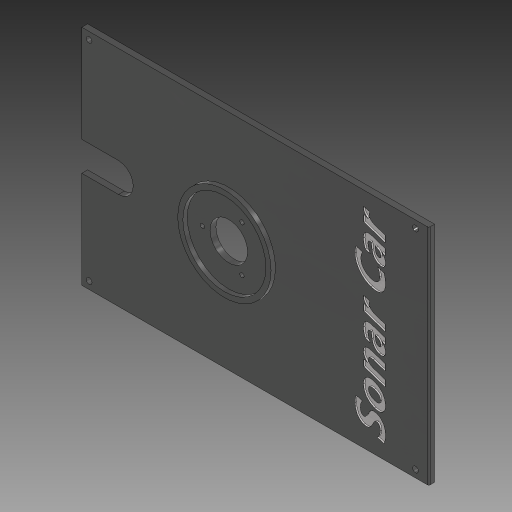
# Autodesk Inventor part: box-top
Saved by Autodesk Inventor 2023 (Build 270158000, 158)
## iProperties
Created: 2024-02-02
Part Number: box-top
Material: Všeobecné
Document SubType Name: Modeling
Designer: matej
Mass: 17.4288 g
Surface Area: 187.276 cm^2
Volume: 17.4288 cm^3
Density: 1 g/cm^3
Appearance: Tmavě šedá
Author: matej
## iProperties of the stored document box-top_3D tisk.ipt
Created: 2024-02-13
Part Number: box-top_3D tisk
Material: Všeobecné
Document SubType Name: Modeling
Designer: zak
Density: 1 g/cm^3
Appearance: Výchozí
Mass: 17.4407 g
Surface Area: 187.376 cm^2
Volume: 17.4407 cm^3
Author: zak
Autodesk Inventor part; units mm, degrees
ref_plane "YZ Plane" through (0, 0, 0) normal (1, 0, 0) x (0, 1, 0)
ref_plane "XZ Plane" through (0, 0, 0) normal (0, 1, 0) x (-1, 0, 0)
ref_plane "XY Plane" through (0, 0, 0) normal (0, 0, 1) x (1, 0, 0)
sketch "Náčrt1" plane through (0, 0, 0) normal (0, 0, 1) x (1, 0, 0)
  line L0 (60, 40) -> (-60, 40)
  line L1 (-60, 40) -> (-60, -40)
  line L2 (-60, -40) -> (60, -40)
  line L3 (60, -40) -> (60, 40)
  line L4 (60, 40) -> (-60, -40) construction
  line L5 (-60, 40) -> (60, -40) construction
  line L6 (58, 38) -> (53, 38)
  line L7 (53, 38) -> (53, 33)
  line L8 (53, 33) -> (58, 33)
  line L9 (58, 33) -> (58, 38)
  line L10 (53, 38) -> (58, 33) construction
  line L11 (58, 38) -> (53, 33) construction
  circle A0 centre (55.5, 35.5) radius 1
  line L12 (58, -33) -> (53, -33)
  line L13 (53, -33) -> (53, -38)
  line L14 (53, -38) -> (58, -38)
  circle A1 centre (55.5, -35.5) radius 1
  line L15 (53, -33) -> (58, -38) construction
  line L16 (58, -33) -> (53, -38) construction
  line L17 (58, -38) -> (58, -33)
  line L18 (-53, 38) -> (-58, 38)
  line L19 (-58, 38) -> (-58, 33)
  line L20 (-58, 33) -> (-53, 33)
  circle A2 centre (-55.5, 35.5) radius 1
  line L21 (-58, 38) -> (-53, 33) construction
  line L22 (-53, 38) -> (-58, 33) construction
  line L23 (-53, 33) -> (-53, 38)
  line L24 (-53, -33) -> (-58, -33)
  line L25 (-58, -33) -> (-58, -38)
  line L26 (-58, -38) -> (-53, -38)
  circle A3 centre (-55.5, -35.5) radius 1
  line L27 (-58, -33) -> (-53, -38) construction
  line L28 (-53, -33) -> (-58, -38) construction
  line L29 (-53, -38) -> (-53, -33)
  line L30 (-58, 38) -> (60, 38)
  line L31 (60, 38) -> (60, -38)
  line L32 (60, -38) -> (-58, -38)
  line L33 (-58, -38) -> (-58, 38)
  point P0 (0, 0)
  dimension "d0" = 120
  dimension "d1" = 80
  dimension "d2" = 5
  dimension "d3" = 5
  dimension "d4" = 2
  dimension "d5" = 2.5
  dimension "d6" = 2
  dimension "d7" = 2
  dimension "d10" = 71
  dimension "d13" = 111
  constraints: 68 end point, 6 parallel, 4 centre point, 4 horizontal, 3 midpoint, 3 perpendicular, 1 point on line, 1 vertical, 39 other
  measures "d0" distance of L0.start L0.end
  measures "d1" distance of L2.end L0.start
  measures "d2" distance of L8.end L7.end
  measures "d3" distance of L7.end L6.end
  measures "d4" diameter of A0
  measures "d5" distance from line of L8 A0.centre
  measures "d6" distance between parallel lines of L0 L6
  measures "d7" distance between parallel lines of L3 L9
  measures "d10" distance of L6.start L12.start
  measures "d13" distance of L6.start L18.start
extrude "Vysunutí1" add sketch "Náčrt1" along normal blind 2 contours L3 L32 L17 L12 L13 L29 L24 L33 L20 L23 L30 L7 L8 L9 | L9 L8 L7 L6 | L14 L13 L12 L17 | L23 L20 L19 L18 | L26 L25 L24 L29
sketch "Náčrt2" plane through (0, 0, 2) normal (0, 0, 1) x (1, 0, 0)
  circle A0 centre (-8, 0) radius 6.4
  line L0 (-58, 38) -> (-58, -38) projected
  point P0 (0, 0)
  dimension "d18" = 12.8
  dimension "d25" = 50
  constraints: 1 centre point
  measures "d18" diameter of A0
  measures "d25" distance from line of L0 A0.centre
extrude "Vysunutí2" cut sketch "Náčrt2" against normal through all
sketch "Náčrt3" plane through (0, 0, 2) normal (0, 0, 1) x (1, 0, 0)
  circle A0 centre (-45.5, 0) radius 5
  line L0 (-58, 38) -> (-58, -38) projected
  line L1 (-70.5, -5) -> (-45.5, -5)
  line L2 (-45.5, -5) -> (-45.5, 5)
  line L3 (-45.5, 5) -> (-70.5, 5)
  line L4 (-70.5, 5) -> (-70.5, -5)
  line L5 (-70.5, -5) -> (-45.5, 5) construction
  line L6 (-45.5, -5) -> (-70.5, 5) construction
  point P0 (0, 0)
  point P1 (-58, 0)
  point P2 (-45.5, -5)
  point P3 (-45.5, 5)
  dimension "d21" = 12.5
  dimension "d22" = 10
  dimension "d43" = 10
  dimension "d44" = 25
  constraints: 12 end point, 3 midpoint, 2 parallel, 1 centre point, 1 horizontal, 1 perpendicular
  measures "d21" distance from line of L0 A0.centre
  measures "d22" diameter of A0
  measures "d43" distance of L1.end L2.end
  measures "d44" distance between parallel lines of L4 L2
extrude "Vysunutí3" cut sketch "Náčrt3" against normal through all
sketch "Náčrt4" plane through (0, 0, 2) normal (0, 0, 1) x (1, 0, 0)
  circle A0 centre (-8, 0) radius 6.4 projected
  circle A1 centre (-8, 0) radius 14.125
  circle A2 centre (-8, 0) radius 15.875
  point P0 (0, 0)
  dimension "d26" = 28.25
  dimension "d27" = 31.75
  constraints: 2 centre point, 2 coincident
  measures "d26" diameter of A1
  measures "d27" diameter of A2
extrude "Vysunutí4" add sketch "Náčrt4" along normal blind 1.5 contours A2
sketch "Náčrt5" plane through (0, 0, 2) normal (0, 0, 1) x (1, 0, 0)
  circle A0 centre (-17, 0) radius 0.75
  circle A1 centre (-8, 0) radius 6.4 projected
  circle A2 centre (-3.5, -7.7942) radius 0.75
  circle A3 centre (-3.5, 7.7942) radius 0.75
  point P0 (0, 0)
  dimension "d31" = 1.5
  dimension "d34" = 360
  dimension "d36" = 9
  constraints: 3 centre point, 2 coincident, 8 other
  measures "d31" diameter of A0
  measures "d36" distance of A1.centre A0.centre
extrude "Vysunutí5" cut sketch "Náčrt5" against normal through all contours A0 | A2 | A3
sketch "Náčrt6" plane through (0, 0, 2) normal (0, 0, 1) x (1, 0, 0)
  line L0 (34.9532, -34.0683) -> (34.9532, 34.0683) construction
  line L1 (34.9532, 34.0683) -> (55, 34.0683) construction
  line L2 (55, 34.0683) -> (55, -34.0683) construction
  line L3 (55, -34.0683) -> (34.9532, -34.0683) construction
  line L4 (60, -38) -> (60, 38) projected
  line L5 (44.7398, -33.252) -> (42.5042, -32.4913)
  spline S0 degree 2 poles (42.5042, -32.4913) (43.0144, -32.0646) (43.5246, -30.8123) (43.5246, -30.0887) knots 0 0 0 1 2 2 2
  spline S1 degree 2 poles (43.5246, -30.0887) (43.5246, -29.662) (43.3669, -28.9756) (43.0979, -28.4561) (42.7268, -28.1221) (42.5135, -28.0479) knots 0 0 0 1 2 3 4 4 4
  spline S2 degree 2 poles (42.5135, -28.0479) (42.2166, -27.9459) (41.7621, -28.1221) (41.3632, -28.5767) (41.0014, -29.2446) (40.8159, -29.6435) knots 0 0 0 1 2 3 4 4 4
  spline S3 degree 2 poles (40.8159, -29.6435) (40.3242, -30.6453) (38.9235, -31.3225) (37.9216, -30.9793) knots 0 0 0 1 2 2 2
  spline S4 degree 2 poles (37.9216, -30.9793) (37.1424, -30.7103) (36.02, -29.7084) (35.2871, -28.3819) (34.9532, -26.842) (34.9532, -26.0442) knots 0 0 0 1 2 3 4 4 4
  spline S5 degree 2 poles (34.9532, -26.0442) (34.9532, -25.265) (35.1387, -24.1147) (35.3335, -23.6787) knots 0 0 0 1 2 2 2
  line L6 (35.3335, -23.6787) -> (37.4207, -24.3837)
  spline S6 degree 2 poles (37.4207, -24.3837) (37.2445, -24.5785) (36.9754, -25.0795) (36.8085, -25.6453) (36.725, -26.239) (36.725, -26.5173) knots 0 0 0 1 2 3 4 4 4
  spline S7 degree 2 poles (36.725, -26.5173) (36.725, -26.9069) (36.8641, -27.5841) (37.1331, -28.1036) (37.5042, -28.4654) (37.7361, -28.5489) knots 0 0 0 1 2 3 4 4 4
  spline S8 degree 2 poles (37.7361, -28.5489) (37.9866, -28.6323) (38.3855, -28.5025) (38.738, -28.1314) (39.0812, -27.547) (39.2574, -27.1759) knots 0 0 0 1 2 3 4 4 4
  spline S9 degree 2 poles (39.2574, -27.1759) (39.5079, -26.6565) (40.0738, -25.8958) (40.7881, -25.4505) (41.7064, -25.4041) (42.3094, -25.6082) knots 0 0 0 1 2 3 4 4 4
  spline S10 degree 2 poles (42.3094, -25.6082) (43.1443, -25.8958) (44.2853, -26.9162) (44.9903, -28.2427) (45.2964, -29.7919) (45.2964, -30.5897) knots 0 0 0 1 2 3 4 4 4
  spline S11 degree 2 poles (45.2964, -30.5897) (45.2964, -31.4153) (45.0181, -32.8067) (44.7398, -33.252) knots 0 0 0 1 2 2 2
  spline S12 degree 2 poles (45.2964, -21.7863) (45.2964, -23.5767) (43.2927, -24.9403) (41.5766, -24.3559) knots 0 0 0 1 2 2 2
  spline S13 degree 2 poles (41.5766, -24.3559) (39.8048, -23.7529) (37.801, -20.9515) (37.801, -19.1426) knots 0 0 0 1 2 2 2
  spline S14 degree 2 poles (37.801, -19.1426) (37.801, -17.3708) (39.8048, -16.0257) (41.4467, -16.5823) knots 0 0 0 1 2 2 2
  spline S15 degree 2 poles (41.4467, -16.5823) (43.2278, -17.1852) (45.2964, -19.9774) (45.2964, -21.7863) knots 0 0 0 1 2 2 2
  spline S16 degree 2 poles (39.4894, -19.7641) (39.4894, -20.5433) (40.5654, -21.7771) (41.5487, -22.111) knots 0 0 0 1 2 2 2
  spline S17 degree 2 poles (41.5487, -22.111) (43.6081, -22.8067) (43.6081, -21.1463) knots 0 0 0 1 1 1
  spline S18 degree 2 poles (43.6081, -21.1463) (43.6081, -19.56) (41.4931, -18.8457) knots 0 0 0 1 1 1
  spline S19 degree 2 poles (41.4931, -18.8457) (39.4894, -18.1685) (39.4894, -19.7641) knots 0 0 0 1 1 1
  line L7 (45.1202, -9.5043) -> (45.1202, -11.7028)
  line L8 (45.1202, -11.7028) -> (41.1498, -10.3578)
  spline S20 degree 2 poles (41.1498, -10.3578) (39.4894, -9.7919) (39.4894, -10.9793) knots 0 0 0 1 1 1
  spline S21 degree 2 poles (39.4894, -10.9793) (39.4894, -11.5451) (40.3706, -12.5841) (41.0478, -12.816) knots 0 0 0 1 2 2 2
  line L9 (41.0478, -12.816) -> (45.1202, -14.1982)
  line L10 (45.1202, -14.1982) -> (45.1202, -16.406)
  line L11 (45.1202, -16.406) -> (37.9773, -13.9756)
  line L12 (37.9773, -13.9756) -> (37.9773, -11.7771)
  line L13 (37.9773, -11.7771) -> (39.109, -12.1574)
  line L14 (39.109, -12.1574) -> (39.109, -12.1296)
  spline S22 degree 2 poles (39.109, -12.1296) (37.801, -10.8958) (37.801, -9.393) knots 0 0 0 1 1 1
  spline S23 degree 2 poles (37.801, -9.393) (37.801, -7.0182) (40.751, -8.0201) knots 0 0 0 1 1 1
  line L15 (40.751, -8.0201) -> (45.1202, -9.5043)
  line L16 (45.1202, -1.8142) -> (45.1202, -3.9014)
  line L17 (45.1202, -3.9014) -> (44.0905, -3.5581)
  line L18 (44.0905, -3.5581) -> (44.0905, -3.586)
  spline S24 degree 2 poles (44.0905, -3.586) (45.2964, -4.7084) (45.2964, -6.1184) knots 0 0 0 1 1 1
  spline S25 degree 2 poles (45.2964, -6.1184) (45.2964, -7.1574) (44.1183, -7.9459) (43.135, -7.6119) knots 0 0 0 1 2 2 2
  spline S26 degree 2 poles (43.135, -7.6119) (41.0571, -6.9069) (40.7324, -4.3374) knots 0 0 0 1 1 1
  line L19 (40.7324, -4.3374) -> (40.4727, -2.3058)
  spline S27 degree 2 poles (40.4727, -2.3058) (39.3038, -1.9162) (39.3038, -3.1778) knots 0 0 0 1 1 1
  spline S28 degree 2 poles (39.3038, -3.1778) (39.3038, -4.458) (40.0645, -5.868) knots 0 0 0 1 1 1
  line L20 (40.0645, -5.868) -> (38.404, -5.3021)
  spline S29 degree 2 poles (38.404, -5.3021) (38.1628, -4.7641) (37.801, -3.0387) (37.801, -2.3893) knots 0 0 0 1 2 2 2
  spline S30 degree 2 poles (37.801, -2.3893) (37.801, 0.6719) (40.853, -0.367) knots 0 0 0 1 1 1
  line L21 (40.853, -0.367) -> (45.1202, -1.8142)
  line L22 (42.2166, -2.8995) -> (41.7343, -2.7418)
  line L23 (41.7343, -2.7418) -> (41.9012, -4.0962)
  spline S31 degree 2 poles (41.9012, -4.0962) (42.0404, -5.2186) (42.8753, -5.4969) knots 0 0 0 1 1 1
  spline S32 degree 2 poles (42.8753, -5.4969) (43.2463, -5.6268) (43.7287, -5.265) (43.7287, -4.8197) knots 0 0 0 1 2 2 2
  spline S33 degree 2 poles (43.7287, -4.8197) (43.7287, -4.1982) (42.8753, -3.1221) (42.2166, -2.8995) knots 0 0 0 1 2 2 2
  spline S34 degree 2 poles (39.9625, 6.3398) (39.7491, 6.0151) (39.7491, 5.4864) knots 0 0 0 1 1 1
  spline S35 degree 2 poles (39.7491, 5.4864) (39.7491, 4.7721) (40.8066, 3.6033) (41.7064, 3.2972) knots 0 0 0 1 2 2 2
  line L24 (41.7064, 3.2972) -> (45.1202, 2.1376)
  line L25 (45.1202, 2.1376) -> (45.1202, -0.0702)
  line L26 (45.1202, -0.0702) -> (37.9773, 2.3602)
  line L27 (37.9773, 2.3602) -> (37.9773, 4.5587)
  line L28 (37.9773, 4.5587) -> (39.3038, 4.1135)
  line L29 (39.3038, 4.1135) -> (39.3038, 4.1413)
  spline S36 degree 2 poles (39.3038, 4.1413) (37.8474, 5.1524) (37.8474, 6.5161) knots 0 0 0 1 1 1
  spline S37 degree 2 poles (37.8474, 6.5161) (37.8474, 6.8686) (37.9309, 7.0356) knots 0 0 0 1 1 1
  line L30 (37.9309, 7.0356) -> (39.9625, 6.3398)
  spline S38 degree 2 poles (44.7676, 17.0634) (45.2964, 15.7925) (45.2964, 14.03) knots 0 0 0 1 1 1
  spline S39 degree 2 poles (45.2964, 14.03) (45.2964, 11.7294) (42.5877, 10.004) (40.3335, 10.774) knots 0 0 0 1 2 2 2
  spline S40 degree 2 poles (40.3335, 10.774) (37.9309, 11.5903) (34.9532, 15.5699) (34.9532, 17.9354) knots 0 0 0 1 2 2 2
  spline S41 degree 2 poles (34.9532, 17.9354) (34.9532, 19.401) (35.315, 20.273) knots 0 0 0 1 1 1
  line L31 (35.315, 20.273) -> (37.4856, 19.5402)
  spline S42 degree 2 poles (37.4856, 19.5402) (36.892, 18.7424) (36.892, 17.453) knots 0 0 0 1 1 1
  spline S43 degree 2 poles (36.892, 17.453) (36.892, 16.043) (38.6638, 13.7146) (40.1758, 13.2044) knots 0 0 0 1 2 2 2
  spline S44 degree 2 poles (40.1758, 13.2044) (41.6229, 12.7035) (43.3484, 13.7517) (43.3484, 15.1339) knots 0 0 0 1 2 2 2
  spline S45 degree 2 poles (43.3484, 15.1339) (43.3484, 16.4511) (42.7083, 17.7684) knots 0 0 0 1 1 1
  line L32 (42.7083, 17.7684) -> (44.7676, 17.0634)
  line L33 (45.1202, 24.4196) -> (45.1202, 22.3324)
  line L34 (45.1202, 22.3324) -> (44.0905, 22.6756)
  line L35 (44.0905, 22.6756) -> (44.0905, 22.6478)
  spline S46 degree 2 poles (44.0905, 22.6478) (45.2964, 21.5254) (45.2964, 20.1153) knots 0 0 0 1 1 1
  spline S47 degree 2 poles (45.2964, 20.1153) (45.2964, 19.0764) (44.1183, 18.2879) (43.135, 18.6218) knots 0 0 0 1 2 2 2
  spline S48 degree 2 poles (43.135, 18.6218) (41.0571, 19.3268) (40.7324, 21.8964) knots 0 0 0 1 1 1
  line L36 (40.7324, 21.8964) -> (40.4727, 23.9279)
  spline S49 degree 2 poles (40.4727, 23.9279) (39.3038, 24.3176) (39.3038, 23.056) knots 0 0 0 1 1 1
  spline S50 degree 2 poles (39.3038, 23.056) (39.3038, 21.7758) (40.0645, 20.3658) knots 0 0 0 1 1 1
  line L37 (40.0645, 20.3658) -> (38.404, 20.9317)
  spline S51 degree 2 poles (38.404, 20.9317) (38.1628, 21.4697) (37.801, 23.1951) (37.801, 23.8445) knots 0 0 0 1 2 2 2
  spline S52 degree 2 poles (37.801, 23.8445) (37.801, 26.9057) (40.853, 25.8667) knots 0 0 0 1 1 1
  line L38 (40.853, 25.8667) -> (45.1202, 24.4196)
  line L39 (42.2166, 23.3343) -> (41.7343, 23.492)
  line L40 (41.7343, 23.492) -> (41.9012, 22.1376)
  spline S53 degree 2 poles (41.9012, 22.1376) (42.0404, 21.0151) (42.8753, 20.7369) knots 0 0 0 1 1 1
  spline S54 degree 2 poles (42.8753, 20.7369) (43.2463, 20.607) (43.7287, 20.9688) (43.7287, 21.414) knots 0 0 0 1 2 2 2
  spline S55 degree 2 poles (43.7287, 21.414) (43.7287, 22.0356) (42.8753, 23.1116) (42.2166, 23.3343) knots 0 0 0 1 2 2 2
  spline S56 degree 2 poles (39.9625, 32.5736) (39.7491, 32.2489) (39.7491, 31.7202) knots 0 0 0 1 1 1
  spline S57 degree 2 poles (39.7491, 31.7202) (39.7491, 31.0059) (40.8066, 29.837) (41.7064, 29.5309) knots 0 0 0 1 2 2 2
  line L41 (41.7064, 29.5309) -> (45.1202, 28.3714)
  line L42 (45.1202, 28.3714) -> (45.1202, 26.1636)
  line L43 (45.1202, 26.1636) -> (37.9773, 28.594)
  line L44 (37.9773, 28.594) -> (37.9773, 30.7925)
  line L45 (37.9773, 30.7925) -> (39.3038, 30.3472)
  line L46 (39.3038, 30.3472) -> (39.3038, 30.3751)
  spline S58 degree 2 poles (39.3038, 30.3751) (37.8474, 31.3862) (37.8474, 32.7498) knots 0 0 0 1 1 1
  spline S59 degree 2 poles (37.8474, 32.7498) (37.8474, 33.1023) (37.9309, 33.2693) knots 0 0 0 1 1 1
  line L47 (37.9309, 33.2693) -> (39.9625, 32.5736)
  point P0 (0, 0)
  point P1 (55, 0)
  point P2 (60, 0)
  dimension "d41" = 5
  constraints: 2 midpoint, 1 horizontal alignment, 2 other
  measures "d41" distance between parallel lines of L4 L2
emboss "Reliéf1" sketch "Náčrt6" operation cut depth 0.5 direction (0, 0, -1)
fillet "Zaoblení2" radius 0.5 1 edges at (60, 0, 2)
